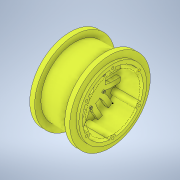
# Autodesk Inventor part: RCT-P009  Rin
Saved by Autodesk Inventor 2020 (Build 240168000, 168)
## iProperties
Created: 2019-09-30
Part Number: RCT-P009  Rin
Material: Genérico
Document SubType Name: Modeling
Designer: david
Density: 1 g/cm^3
Appearance: Valor por defecto
Author: david
Autodesk Inventor part; units mm, degrees
ref_plane "YZ Plane" through (0, 0, 0) normal (1, 0, 0) x (0, 1, 0)
sketch "Boceto1" plane through (0, 0, 0) normal (0, 0, 1) x (1, 0, 0)
  line L0 (0, 0) -> (22.088, 0) construction
  line L1 (12.2099, 0) -> (37.3099, 0) construction
  line L2 (0, 0) -> (0, 21.5) construction
  line L3 (0, 0) -> (21.5, 0) construction
  line L4 (0, 21.5) -> (32.3, 21.5)
  line L5 (0, 21.5) -> (32.3, 21.5) construction
  line L6 (32.3, 21.5) -> (32.3, 28.5)
  line L7 (32.3, 28.5) -> (26.8, 28.5)
  line L8 (0, 21.5) -> (0, 28.5)
  line L9 (0, 21.5) -> (7, 21.5) construction
  line L10 (0, 28.5) -> (5.5, 28.5)
  line L11 (5.5, 28.5) -> (5.5, 24.1)
  line L12 (5.5, 24.1) -> (26.8, 24.1)
  line L13 (26.8, 24.1) -> (26.8, 28.5)
  dimension "d14" = 21.5
  dimension "d15" = 90
  dimension "d16" = 32.3
  dimension "d17" = 0
  dimension "d18" = 7
  dimension "d19" = 5.5
  dimension "d20" = 7
  dimension "d21" = 90
  dimension "d23" = 5.5
  dimension "d24" = 4.4
  constraints: 28 end point, 8 horizontal, 4 perpendicular, 3 equal length, 2 vertical, 1 point on line
  measures "d14" distance of L0.start L2.end
  measures "d15" angle of L3 L2
  measures "d16" distance of L2.end L4.end
  measures "d17" distance between parallel lines of L4 L5
  measures "d18" distance of L4.end L6.end
  measures "d19" distance of L6.end L7.end
  measures "d20" distance of L2.end L8.end
  measures "d21" angle of L9 L8
  measures "d23" distance of L8.end L10.end
  measures "d24" distance of L10.end L11.end
revolve "Revolución1" add sketch "Boceto1" angle 360 about axis through (12.2099, 0, 0) along (1, 0, 0)
ref_plane "Plano de trabajo1" through (16.5, 0, 0) normal (-1, 0, 0) x (0, 0, 1)
sketch "Boceto2" plane through (16.5, 0, 0) normal (-1, 0, 0) x (0, 0, 1)
  point P0 (0, 0)
  point P1 (0, 0)
sketch "Boceto12" plane through (16.5, 0, 0) normal (-1, 0, 0) x (0, 0, 1)
  circle A0 centre (0, 0) radius 10.45
  dimension "d56" = 20.9
  constraints: 1 centre point, 1 coincident
  measures "d56" diameter of A0
extrude "Extrusión10" add sketch "Boceto12" along normal blind 4
sketch "Boceto13" plane through (12.5, 0, 0) normal (-1, 0, 0) x (0, 0, 1)
  circle A0 centre (0, 0) radius 8.8
  dimension "d59" = 17.6
  constraints: 1 centre point, 1 coincident
  measures "d59" diameter of A0
extrude "Extrusión11" add sketch "Boceto13" along normal blind 4.2
sketch "Boceto14" plane through (8.3, 0, 0) normal (-1, 0, 0) x (0, 0, 1)
  line L0 (0, 6.8127) -> (5.9, 3.4064)
  line L1 (5.9, 3.4064) -> (5.9, -3.4064)
  line L2 (5.9, -3.4064) -> (0, -6.8127)
  line L3 (0, -6.8127) -> (-5.9, -3.4064)
  line L4 (-5.9, -3.4064) -> (-5.9, 3.4064)
  line L5 (-5.9, 3.4064) -> (0, 6.8127)
  point P0 (0, 0)
  point P1 (0, 0)
  dimension "d62" = 11.8
  constraints: 12 end point, 1 coincident, 13 other
  measures "d62" distance between parallel lines of L1 L4
extrude "Extrusión12" cut sketch "Boceto14" against normal blind 4
sketch "Boceto15" plane through (12.3, 0, 0) normal (-1, 0, 0) x (0, 0, 1)
  circle A0 centre (0, 0) radius 4.5
  dimension "d65" = 9
  constraints: 1 centre point, 1 coincident
  measures "d65" diameter of A0
extrude "Extrusión13" cut sketch "Boceto15" against normal blind 1
sketch "Boceto16" plane through (13.3, 0, 0) normal (-1, 0, 0) x (0, 0, 1)
  circle A0 centre (0, 0) radius 3.5
  dimension "d68" = 7
  constraints: 1 centre point, 1 coincident
  measures "d68" diameter of A0
extrude "Extrusión14" cut sketch "Boceto16" against normal blind 2.1
sketch "Boceto17" plane through (15.4, 0, 0) normal (-1, 0, 0) x (0, 0, 1)
  circle A0 centre (0, 0) radius 2.5
  dimension "d71" = 5
  constraints: 1 centre point, 1 coincident
  measures "d71" diameter of A0
extrude "Extrusión15" cut sketch "Boceto17" against normal blind 2.1
ref_plane "Plano de trabajo2" through (12.5, 0, 0) normal (-1, 0, 0) x (0, 0, 1)
sketch "Boceto20" plane through (12.5, 0, 0) normal (-1, 0, 0) x (0, 0, 1)
  line L0 (0.0673, 12.0664) -> (10.4835, 5.9749) construction
  line L1 (10.4835, 5.9749) -> (10.4162, -6.0915) construction
  line L2 (10.4162, -6.0915) -> (-0.0673, -12.0664) construction
  line L3 (-0.0673, -12.0664) -> (-10.4835, -5.9749) construction
  line L4 (-10.4835, -5.9749) -> (-10.4162, 6.0915) construction
  line L5 (-10.4162, 6.0915) -> (0.0673, 12.0664) construction
  circle A0 centre (0, 0) radius 10.45
  line L6 (0.0673, 12.0664) -> (-0.9327, 12.0664)
  line L7 (-0.9327, 12.0664) -> (-1.9587, 14.8855)
  circle A1 centre (0, 0) radius 21.5
  line L8 (0, 21.5) -> (0, 20.8746) construction
  line L9 (-1.9587, 14.8855) -> (-5.3823, 20.8154)
  line L10 (-1.9587, 14.8855) -> (4.8885, 14.8855) construction
  line L11 (-8.5615, 19.7218) -> (-4.961, 13.4855)
  line L12 (-4.961, 13.4855) -> (-3.6205, 9.8028)
  line L13 (0, 8.7664) -> (0.0673, 8.7664)
  line L14 (1.9587, 14.8855) -> (5.3823, 20.8154)
  line L15 (0.9327, 12.0664) -> (1.9587, 14.8855)
  line L16 (8.5615, 19.7218) -> (4.961, 13.4855)
  line L17 (4.961, 13.4855) -> (3.6205, 9.8028)
  line L18 (-0.0673, 12.0664) -> (0.9327, 12.0664)
  line L19 (-21.3604, 2.4464) -> (-14.1593, 2.4464)
  line L20 (-14.1593, 2.4464) -> (-10.2997, 1.7659)
  line L21 (-10.9162, 5.2255) -> (-13.8706, 5.7464)
  line L22 (-13.8706, 5.7464) -> (-20.7178, 5.7464)
  line L23 (-10.4162, 6.0915) -> (-10.9162, 5.2255)
  line L24 (-10.4835, 5.9749) -> (-9.9835, 6.8409)
  line L25 (-9.9835, 6.8409) -> (-11.9119, 9.1391)
  line L26 (-11.9119, 9.1391) -> (-15.3355, 15.0689)
  line L27 (-12.7989, 17.2754) -> (-9.1983, 11.0391)
  line L28 (-9.1983, 11.0391) -> (-6.6792, 8.0369)
  line L29 (-12.7989, -17.2754) -> (-9.1983, -11.0391)
  line L30 (-9.1983, -11.0391) -> (-6.6792, -8.0369)
  line L31 (-9.9835, -6.8409) -> (-11.9119, -9.1391)
  line L32 (-11.9119, -9.1391) -> (-15.3355, -15.0689)
  line L33 (-10.4835, -5.9749) -> (-9.9835, -6.8409)
  line L34 (-10.4162, -6.0915) -> (-10.9162, -5.2255)
  line L35 (-10.9162, -5.2255) -> (-13.8706, -5.7464)
  line L36 (-13.8706, -5.7464) -> (-20.7178, -5.7464)
  line L37 (-21.3604, -2.4464) -> (-14.1593, -2.4464)
  line L38 (-14.1593, -2.4464) -> (-10.2997, -1.7659)
  line L39 (8.5615, -19.7218) -> (4.961, -13.4855)
  line L40 (4.961, -13.4855) -> (3.6205, -9.8028)
  line L41 (0.9327, -12.0664) -> (1.9587, -14.8855)
  line L42 (1.9587, -14.8855) -> (5.3823, -20.8154)
  line L43 (-0.0673, -12.0664) -> (0.9327, -12.0664)
  line L44 (0.0673, -12.0664) -> (-0.9327, -12.0664)
  line L45 (-0.9327, -12.0664) -> (-1.9587, -14.8855)
  line L46 (-1.9587, -14.8855) -> (-5.3823, -20.8154)
  line L47 (-8.5615, -19.7218) -> (-4.961, -13.4855)
  line L48 (-4.961, -13.4855) -> (-3.6205, -9.8028)
  line L49 (21.3604, -2.4464) -> (14.1593, -2.4464)
  line L50 (14.1593, -2.4464) -> (10.2997, -1.7659)
  line L51 (10.9162, -5.2255) -> (13.8706, -5.7464)
  line L52 (13.8706, -5.7464) -> (20.7178, -5.7464)
  line L53 (10.4162, -6.0915) -> (10.9162, -5.2255)
  line L54 (10.4835, -5.9749) -> (9.9835, -6.8409)
  line L55 (9.9835, -6.8409) -> (11.9119, -9.1391)
  line L56 (11.9119, -9.1391) -> (15.3355, -15.0689)
  line L57 (12.7989, -17.2754) -> (9.1983, -11.0391)
  line L58 (9.1983, -11.0391) -> (6.6792, -8.0369)
  line L59 (12.7989, 17.2754) -> (9.1983, 11.0391)
  line L60 (9.1983, 11.0391) -> (6.6792, 8.0369)
  line L61 (9.9835, 6.8409) -> (11.9119, 9.1391)
  line L62 (11.9119, 9.1391) -> (15.3355, 15.0689)
  line L63 (10.4835, 5.9749) -> (9.9835, 6.8409)
  line L64 (10.4162, 6.0915) -> (10.9162, 5.2255)
  line L65 (10.9162, 5.2255) -> (13.8706, 5.7464)
  line L66 (13.8706, 5.7464) -> (20.7178, 5.7464)
  line L67 (21.3604, 2.4464) -> (14.1593, 2.4464)
  line L68 (14.1593, 2.4464) -> (10.2997, 1.7659)
  arc A2 (21.3604, 2.4464) -> (12.7989, 17.2754) centre (0, 0) ccw
  arc A3 (8.5615, 19.7218) -> (-8.5615, 19.7218) centre (0, 0) ccw
  arc A4 (-12.7989, 17.2754) -> (-21.3604, 2.4464) centre (0, 0) ccw
  arc A5 (-21.3604, -2.4464) -> (-12.7989, -17.2754) centre (0, 0) ccw
  arc A6 (-21.3604, -2.4464) -> (-12.7989, -17.2754) centre (0, 0) ccw
  arc A7 (-12.7989, 17.2754) -> (-21.3604, 2.4464) centre (0, 0) ccw
  arc A8 (8.5615, 19.7218) -> (-8.5615, 19.7218) centre (0, 0) ccw
  arc A9 (21.3604, 2.4464) -> (12.7989, 17.2754) centre (0, 0) ccw
  arc A10 (-8.5615, -19.7218) -> (8.5615, -19.7218) centre (0, 0) ccw
  arc A11 (12.7989, -17.2754) -> (21.3604, -2.4464) centre (0, 0) ccw
  arc A12 (-8.5615, -19.7218) -> (8.5615, -19.7218) centre (0, 0) ccw
  arc A13 (12.7989, -17.2754) -> (21.3604, -2.4464) centre (0, 0) ccw
  arc A14 (3.6205, 9.8028) -> (-3.6205, 9.8028) centre (0, 0) ccw
  arc A15 (-6.6792, 8.0369) -> (-10.2997, 1.7659) centre (0, 0) ccw
  arc A16 (-10.2997, -1.7659) -> (-6.6792, -8.0369) centre (0, 0) ccw
  arc A17 (-3.6205, -9.8028) -> (3.6205, -9.8028) centre (0, 0) ccw
  arc A18 (6.6792, -8.0369) -> (10.2997, -1.7659) centre (0, 0) ccw
  arc A19 (10.2997, 1.7659) -> (6.6792, 8.0369) centre (0, 0) ccw
  dimension "d107" = 1
  dimension "d108" = 3
  dimension "d109" = 120
  dimension "d110" = 3.3
  dimension "d111" = 360
  dimension "d114" = 5.9299
  dimension "d115" = 3.02
  constraints: 138 end point, 38 point on circle, 19 centre point, 7 symmetric about line, 4 coincident, 3 parallel, 2 horizontal, 1 concentric, 1 equal length, 1 point on line, 1 vertical, 163 other
  measures "d107" distance of L6.start L6.end
  measures "d108" distance of L6.end L10.start
  measures "d109" angle of L10 L9
  measures "d110" distance between parallel lines of L9 L11
  measures "d114" vertical distance of L14.start L14.end
  measures "d115" distance from line of L13.end L66
extrude "Extrusión16" add sketch "Boceto20" against normal blind 4 contours A0 L60 L59 A1 L62 L61 L63 L64 L65 L66 L67 L68 | L50 L49 A1 L52 L51 L53 L54 L55 L56 L57 L58 A0 | A0 L12 L11 A1 L9 L7 L6 L18 L15 L14 L16 L17 | L40 L39 A1 L42 L41 L43 L44 L45 L46 L47 L48 A0 | L66 L65 L64 L63 L61 L62 A1 | A1 L56 L55 L54 L53 L51 L52 | A0 L20 L19 A1 L22 L21 L23 L24 L25 L26 L27 L28 | L30 L29 A1 L32 L31 L33 L34 L35 L36 L37 L38 A0 | L14 L15 L18 L6 L7 L9 A1 | A1 L46 L45 L44 L43 L41 L42 | L26 L25 L24 L23 L21 L22 A1 | A1 L36 L35 L34 L33 L31 L32
sketch "Boceto22" plane through (16.5, 0, 0) normal (1, 0, 0) x (0, 0, -1)
  line L0 (1.9587, 14.8855) -> (5.3823, 20.8154)
  line L1 (0.9327, 12.0664) -> (1.9587, 14.8855)
  line L2 (-0.0673, 12.0664) -> (0.9327, 12.0664)
  line L3 (0, 21.5) -> (0, 20.8746) construction
  line L4 (0.0673, 12.0664) -> (-0.9327, 12.0664)
  line L5 (-1.9587, 14.8855) -> (4.8885, 14.8855) construction
  line L6 (-0.9327, 12.0664) -> (-1.9587, 14.8855)
  line L7 (-1.9587, 14.8855) -> (-5.3823, 20.8154)
  arc A0 (5.3823, 20.8154) -> (-5.3823, 20.8154) centre (0, 0) ccw
  circle A1 centre (0, 0) radius 21.5 projected
  line L8 (-5.3823, 20.8154) -> (-1.9587, 14.8855)
  line L9 (-0.9327, 12.0664) -> (0.9327, 12.0664)
  line L10 (1.9587, 14.8855) -> (5.3823, 20.8154)
  line L11 (-10.4835, 5.9749) -> (-9.9835, 6.8409)
  line L12 (-10.4162, 6.0915) -> (-10.9162, 5.2255)
  line L13 (-10.9162, 5.2255) -> (-9.9835, 6.8409)
  line L14 (-9.9835, 6.8409) -> (-11.9119, 9.1391)
  line L15 (-10.9162, 5.2255) -> (-13.8706, 5.7464)
  line L16 (-13.8706, 5.7464) -> (-10.447, 11.6763) construction
  line L17 (-11.9119, 9.1391) -> (-15.3355, 15.0689)
  line L18 (-11.9119, 9.1391) -> (-15.3355, 15.0689)
  line L19 (-13.8706, 5.7464) -> (-20.7178, 5.7464)
  line L20 (-20.7178, 5.7464) -> (-13.8706, 5.7464)
  arc A2 (-15.3355, 15.0689) -> (-20.7178, 5.7464) centre (0, 0) ccw
  line L21 (-18.6195, 10.75) -> (-18.0779, 10.4373) construction
  line L22 (-10.4162, -6.0915) -> (-10.9162, -5.2255)
  line L23 (-10.4835, -5.9749) -> (-9.9835, -6.8409)
  line L24 (-9.9835, -6.8409) -> (-10.9162, -5.2255)
  line L25 (-10.9162, -5.2255) -> (-13.8706, -5.7464)
  line L26 (-9.9835, -6.8409) -> (-11.9119, -9.1391)
  line L27 (-11.9119, -9.1391) -> (-15.3355, -3.2092) construction
  line L28 (-13.8706, -5.7464) -> (-20.7178, -5.7464)
  line L29 (-13.8706, -5.7464) -> (-20.7178, -5.7464)
  line L30 (-11.9119, -9.1391) -> (-15.3355, -15.0689)
  line L31 (-15.3355, -15.0689) -> (-11.9119, -9.1391)
  arc A3 (-20.7178, -5.7464) -> (-15.3355, -15.0689) centre (0, 0) ccw
  line L32 (-18.6195, -10.75) -> (-18.0779, -10.4373) construction
  line L33 (0.0673, -12.0664) -> (-0.9327, -12.0664)
  line L34 (-0.0673, -12.0664) -> (0.9327, -12.0664)
  line L35 (0.9327, -12.0664) -> (-0.9327, -12.0664)
  line L36 (-0.9327, -12.0664) -> (-1.9587, -14.8855)
  line L37 (0.9327, -12.0664) -> (1.9587, -14.8855)
  line L38 (1.9587, -14.8855) -> (-4.8885, -14.8855) construction
  line L39 (-1.9587, -14.8855) -> (-5.3823, -20.8154)
  line L40 (-1.9587, -14.8855) -> (-5.3823, -20.8154)
  line L41 (1.9587, -14.8855) -> (5.3823, -20.8154)
  line L42 (5.3823, -20.8154) -> (1.9587, -14.8855)
  arc A4 (-5.3823, -20.8154) -> (5.3823, -20.8154) centre (0, 0) ccw
  line L43 (0, -21.5) -> (0, -20.8746) construction
  line L44 (10.4835, -5.9749) -> (9.9835, -6.8409)
  line L45 (10.4162, -6.0915) -> (10.9162, -5.2255)
  line L46 (10.9162, -5.2255) -> (9.9835, -6.8409)
  line L47 (9.9835, -6.8409) -> (11.9119, -9.1391)
  line L48 (10.9162, -5.2255) -> (13.8706, -5.7464)
  line L49 (13.8706, -5.7464) -> (10.447, -11.6763) construction
  line L50 (11.9119, -9.1391) -> (15.3355, -15.0689)
  line L51 (11.9119, -9.1391) -> (15.3355, -15.0689)
  line L52 (13.8706, -5.7464) -> (20.7178, -5.7464)
  line L53 (20.7178, -5.7464) -> (13.8706, -5.7464)
  arc A5 (15.3355, -15.0689) -> (20.7178, -5.7464) centre (0, 0) ccw
  line L54 (18.6195, -10.75) -> (18.0779, -10.4373) construction
  line L55 (10.4162, 6.0915) -> (10.9162, 5.2255)
  line L56 (10.4835, 5.9749) -> (9.9835, 6.8409)
  line L57 (9.9835, 6.8409) -> (10.9162, 5.2255)
  line L58 (10.9162, 5.2255) -> (13.8706, 5.7464)
  line L59 (9.9835, 6.8409) -> (11.9119, 9.1391)
  line L60 (11.9119, 9.1391) -> (15.3355, 3.2092) construction
  line L61 (13.8706, 5.7464) -> (20.7178, 5.7464)
  line L62 (13.8706, 5.7464) -> (20.7178, 5.7464)
  line L63 (11.9119, 9.1391) -> (15.3355, 15.0689)
  line L64 (15.3355, 15.0689) -> (11.9119, 9.1391)
  arc A6 (20.7178, 5.7464) -> (15.3355, 15.0689) centre (0, 0) ccw
  line L65 (18.6195, 10.75) -> (18.0779, 10.4373) construction
  point P0 (4.961, 13.4855)
  point P1 (0, 8.7664)
  point P2 (-4.961, 13.4855)
  point P3 (-7.592, 4.3832)
  point P4 (-9.1983, 11.0391)
  point P5 (-14.1593, 2.4464)
  point P6 (-7.592, -4.3832)
  point P7 (-14.1593, -2.4464)
  point P8 (-9.1983, -11.0391)
  point P9 (0, -8.7664)
  point P10 (-4.961, -13.4855)
  point P11 (4.961, -13.4855)
  point P12 (7.592, -4.3832)
  point P13 (9.1983, -11.0391)
  point P14 (14.1593, -2.4464)
  point P15 (7.592, 4.3832)
  point P16 (14.1593, 2.4464)
  point P17 (9.1983, 11.0391)
  dimension "d116" = 1
  dimension "d117" = 3
  dimension "d118" = 120
  dimension "d119" = 5.9299
  dimension "d120" = 170
  dimension "d121" = 5.3823
  dimension "d122" = 3.3
  dimension "d123" = 1.4
  dimension "d124" = 5.0036
  dimension "d125" = 4.6908
  dimension "d126" = 1.3632
  dimension "d129" = 360
  constraints: 132 end point, 12 point on circle, 6 centre point, 6 point on line, 5 symmetric about line, 3 horizontal, 1 coincident, 1 collinear, 1 concentric, 1 equal length, 1 parallel, 1 vertical, 163 other
  measures "d116" distance of L4.start L4.end
  measures "d117" distance of L4.end L5.start
  measures "d118" angle of L5 L7
  measures "d119" vertical distance of L1.end L0.end
  measures "d120" angle of L1 L10
  measures "d121" distance from line of L0.end L3
  measures "d122" distance from line of point (4.961, 13.486) L10
  measures "d123" distance from line of point (4.961, 13.486) L5
  measures "d124" distance from line of L3.start L10
  measures "d125" distance from line of L3.end L10
  measures "d126" distance from line of point (0, 8.766) L10
extrude "Extrusión17" cut sketch "Boceto22" against normal blind 2 contours L1 L2 L4 L6 L7 A0 L0 | A1 L61 L58 L55 L56 L59 L63 | L17 L14 L11 L12 L15 L19 A1 | L28 L25 L22 L23 L26 L30 A1 | A1 L50 L47 L44 L45 L48 L52 | L39 L36 L33 L34 L37 L41 A1
sketch "Boceto23" plane through (32.3, 0, 0) normal (1, 0, 0) x (0, 0, -1)
  circle A0 centre (0, 0) radius 28.5
  circle A1 centre (0, 0) radius 26
  circle A2 centre (0, 0) radius 24
  dimension "d133" = 2.5
  dimension "d134" = 2
  dimension "d135" = 57
  constraints: 3 centre point, 1 coincident
  measures "d133" radial gap between concentric circles of A0 A1
  measures "d134" radial gap between concentric circles of A1 A2
  measures "d135" diameter of A0
extrude "Extrusión18" cut sketch "Boceto23" against normal blind 2 contours A1
sketch "Boceto24" plane through (0, 0, 0) normal (-1, 0, 0) x (0, 0, 1)
  circle A0 centre (0, 0) radius 28.5
  circle A1 centre (0, 0) radius 28.5 projected
  circle A2 centre (0, 0) radius 26
  circle A3 centre (0, 0) radius 24
  dimension "d138" = 2.5
  dimension "d139" = 2
  constraints: 3 centre point, 1 coincident, 1 concentric
  measures "d138" radial gap between concentric circles of A0 A2
  measures "d139" radial gap between concentric circles of A2 A3
extrude "Extrusión19" cut sketch "Boceto24" against normal blind 2 contours A2
sketch "Boceto28" plane through (12.5, 0, 0) normal (-1, 0, 0) x (0, 0, 1)
  line L0 (8.5615, -19.7218) -> (4.961, -13.4855)
  line L1 (4.961, -13.4855) -> (3.6205, -9.8028)
  line L2 (-0.0673, -12.0664) -> (0.9327, -12.0664)
  line L3 (0.0673, -12.0664) -> (-0.9327, -12.0664)
  line L4 (0.9327, -12.0664) -> (1.9587, -14.8855)
  arc A0 (-3.6205, -9.8028) -> (3.6205, -9.8028) centre (0, 0) ccw
  line L5 (-0.9327, -12.0664) -> (-1.9587, -14.8855)
  line L6 (-4.961, -13.4855) -> (-3.6205, -9.8028)
  line L7 (1.9587, -14.8855) -> (5.3823, -20.8154)
  line L8 (-1.9587, -14.8855) -> (-5.3823, -20.8154)
  line L9 (-8.5615, -19.7218) -> (-4.961, -13.4855)
  line L10 (4.961, -13.4855) -> (8.5615, -19.7218) projected
  line L11 (3.6205, -9.8028) -> (4.961, -13.4855) projected
  line L12 (8.5615, -19.7218) -> (4.961, -13.4855)
  line L13 (4.961, -13.4855) -> (3.6205, -9.8028)
  arc A1 (-5.3823, -20.8154) -> (5.3823, -20.8154) centre (0, 0) ccw projected
  line L14 (5.3823, -20.8154) -> (1.9587, -14.8855)
  line L15 (1.9587, -14.8855) -> (0.9327, -12.0664) projected
  line L16 (0.9327, -12.0664) -> (-0.9327, -12.0664)
  line L17 (-1.9587, -14.8855) -> (-5.3823, -20.8154)
  line L18 (-8.5615, -19.7218) -> (-4.961, -13.4855)
  arc A2 (-3.6205, -9.8028) -> (3.6205, -9.8028) centre (0, 0) ccw
  circle A3 centre (0, 0) radius 21.5 projected
  arc A4 (-8.5615, -19.7218) -> (-5.3823, -20.8154) centre (0, 0) ccw
  arc A5 (5.3823, -20.8154) -> (8.5615, -19.7218) centre (0, 0) ccw
  arc A6 (-8.5615, -19.7218) -> (-5.3823, -20.8154) centre (0, 0) ccw
  arc A7 (5.3823, -20.8154) -> (8.5615, -19.7218) centre (0, 0) ccw
  arc A8 (5.3823, -20.8154) -> (8.5615, -19.7218) centre (0, 0) ccw
  arc A9 (-8.5615, -19.7218) -> (-5.3823, -20.8154) centre (0, 0) ccw
  arc A10 (-6.6792, -8.0369) -> (-3.6205, -9.8028) centre (0, 0) ccw projected
  line L19 (-4.961, -13.4855) -> (-3.6205, -9.8028) projected
  line L20 (-3.6205, -9.8028) -> (-4.961, -13.4855)
  line L21 (-8.5615, -19.7218) -> (-4.961, -13.4855) projected
  line L22 (-4.961, -13.4855) -> (-8.5615, -19.7218)
  line L23 (10.4835, -5.9749) -> (9.9835, -6.8409)
  line L24 (10.4162, -6.0915) -> (10.9162, -5.2255)
  line L25 (10.9162, -5.2255) -> (9.9835, -6.8409)
  line L26 (9.1983, -11.0391) -> (6.6792, -8.0369)
  line L27 (6.6792, -8.0369) -> (9.1983, -11.0391)
  arc A11 (6.6792, -8.0369) -> (10.2997, -1.7659) centre (0, 0) ccw
  arc A12 (6.6792, -8.0369) -> (10.2997, -1.7659) centre (0, 0) ccw
  line L28 (9.9835, -6.8409) -> (11.9119, -9.1391)
  line L29 (10.9162, -5.2255) -> (13.8706, -5.7464)
  line L30 (14.1593, -2.4464) -> (10.2997, -1.7659)
  line L31 (13.8706, -5.7464) -> (20.7178, -5.7464)
  line L32 (20.7178, -5.7464) -> (13.8706, -5.7464)
  line L33 (21.3604, -2.4464) -> (14.1593, -2.4464)
  line L34 (21.3604, -2.4464) -> (14.1593, -2.4464)
  line L35 (14.1593, -2.4464) -> (10.2997, -1.7659)
  line L36 (11.9119, -9.1391) -> (15.3355, -15.0689)
  line L37 (11.9119, -9.1391) -> (15.3355, -15.0689)
  line L38 (12.7989, -17.2754) -> (9.1983, -11.0391)
  line L39 (9.1983, -11.0391) -> (12.7989, -17.2754)
  arc A13 (12.7989, -17.2754) -> (15.3355, -15.0689) centre (0, 0) ccw
  line L40 (12.7989, -17.2754) -> (9.1983, -11.0391)
  arc A14 (20.7178, -5.7464) -> (21.3604, -2.4464) centre (0, 0) ccw
  arc A15 (12.7989, -17.2754) -> (15.3355, -15.0689) centre (0, 0) ccw
  arc A16 (12.7989, -17.2754) -> (15.3355, -15.0689) centre (0, 0) ccw
  arc A17 (20.7178, -5.7464) -> (21.3604, -2.4464) centre (0, 0) ccw
  arc A18 (20.7178, -5.7464) -> (21.3604, -2.4464) centre (0, 0) ccw
  line L41 (10.4162, 6.0915) -> (10.9162, 5.2255)
  line L42 (10.4835, 5.9749) -> (9.9835, 6.8409)
  line L43 (9.9835, 6.8409) -> (10.9162, 5.2255)
  line L44 (14.1593, 2.4464) -> (10.2997, 1.7659)
  line L45 (10.2997, 1.7659) -> (14.1593, 2.4464)
  arc A19 (10.2997, 1.7659) -> (6.6792, 8.0369) centre (0, 0) ccw
  arc A20 (10.2997, 1.7659) -> (6.6792, 8.0369) centre (0, 0) ccw
  line L46 (10.9162, 5.2255) -> (13.8706, 5.7464)
  line L47 (9.9835, 6.8409) -> (11.9119, 9.1391)
  line L48 (9.1983, 11.0391) -> (6.6792, 8.0369)
  line L49 (11.9119, 9.1391) -> (15.3355, 15.0689)
  line L50 (15.3355, 15.0689) -> (11.9119, 9.1391)
  line L51 (12.7989, 17.2754) -> (9.1983, 11.0391)
  line L52 (12.7989, 17.2754) -> (9.1983, 11.0391)
  line L53 (9.1983, 11.0391) -> (6.6792, 8.0369)
  line L54 (13.8706, 5.7464) -> (20.7178, 5.7464)
  line L55 (13.8706, 5.7464) -> (20.7178, 5.7464)
  line L56 (21.3604, 2.4464) -> (14.1593, 2.4464)
  line L57 (14.1593, 2.4464) -> (21.3604, 2.4464)
  arc A21 (21.3604, 2.4464) -> (20.7178, 5.7464) centre (0, 0) ccw
  line L58 (21.3604, 2.4464) -> (14.1593, 2.4464)
  arc A22 (15.3355, 15.0689) -> (12.7989, 17.2754) centre (0, 0) ccw
  arc A23 (21.3604, 2.4464) -> (20.7178, 5.7464) centre (0, 0) ccw
  arc A24 (21.3604, 2.4464) -> (20.7178, 5.7464) centre (0, 0) ccw
  arc A25 (15.3355, 15.0689) -> (12.7989, 17.2754) centre (0, 0) ccw
  arc A26 (15.3355, 15.0689) -> (12.7989, 17.2754) centre (0, 0) ccw
  line L59 (-0.0673, 12.0664) -> (0.9327, 12.0664)
  line L60 (0.0673, 12.0664) -> (-0.9327, 12.0664)
  line L61 (-0.9327, 12.0664) -> (0.9327, 12.0664)
  line L62 (4.961, 13.4855) -> (3.6205, 9.8028)
  line L63 (3.6205, 9.8028) -> (4.961, 13.4855)
  arc A27 (3.6205, 9.8028) -> (-3.6205, 9.8028) centre (0, 0) ccw
  arc A28 (3.6205, 9.8028) -> (-3.6205, 9.8028) centre (0, 0) ccw
  line L64 (0.9327, 12.0664) -> (1.9587, 14.8855)
  line L65 (-0.9327, 12.0664) -> (-1.9587, 14.8855)
  line L66 (-4.961, 13.4855) -> (-3.6205, 9.8028)
  line L67 (-1.9587, 14.8855) -> (-5.3823, 20.8154)
  line L68 (-5.3823, 20.8154) -> (-1.9587, 14.8855)
  line L69 (-8.5615, 19.7218) -> (-4.961, 13.4855)
  line L70 (-8.5615, 19.7218) -> (-4.961, 13.4855)
  line L71 (-4.961, 13.4855) -> (-3.6205, 9.8028)
  line L72 (1.9587, 14.8855) -> (5.3823, 20.8154)
  line L73 (1.9587, 14.8855) -> (5.3823, 20.8154)
  line L74 (8.5615, 19.7218) -> (4.961, 13.4855)
  line L75 (4.961, 13.4855) -> (8.5615, 19.7218)
  arc A29 (8.5615, 19.7218) -> (5.3823, 20.8154) centre (0, 0) ccw
  line L76 (8.5615, 19.7218) -> (4.961, 13.4855)
  arc A30 (-5.3823, 20.8154) -> (-8.5615, 19.7218) centre (0, 0) ccw
  arc A31 (8.5615, 19.7218) -> (5.3823, 20.8154) centre (0, 0) ccw
  arc A32 (8.5615, 19.7218) -> (5.3823, 20.8154) centre (0, 0) ccw
  arc A33 (-5.3823, 20.8154) -> (-8.5615, 19.7218) centre (0, 0) ccw
  arc A34 (-5.3823, 20.8154) -> (-8.5615, 19.7218) centre (0, 0) ccw
  line L77 (-10.4835, 5.9749) -> (-9.9835, 6.8409)
  line L78 (-10.4162, 6.0915) -> (-10.9162, 5.2255)
  line L79 (-10.9162, 5.2255) -> (-9.9835, 6.8409)
  line L80 (-9.1983, 11.0391) -> (-6.6792, 8.0369)
  line L81 (-6.6792, 8.0369) -> (-9.1983, 11.0391)
  arc A35 (-6.6792, 8.0369) -> (-10.2997, 1.7659) centre (0, 0) ccw
  arc A36 (-6.6792, 8.0369) -> (-10.2997, 1.7659) centre (0, 0) ccw
  line L82 (-9.9835, 6.8409) -> (-11.9119, 9.1391)
  line L83 (-10.9162, 5.2255) -> (-13.8706, 5.7464)
  line L84 (-14.1593, 2.4464) -> (-10.2997, 1.7659)
  line L85 (-13.8706, 5.7464) -> (-20.7178, 5.7464)
  line L86 (-20.7178, 5.7464) -> (-13.8706, 5.7464)
  line L87 (-21.3604, 2.4464) -> (-14.1593, 2.4464)
  line L88 (-21.3604, 2.4464) -> (-14.1593, 2.4464)
  line L89 (-14.1593, 2.4464) -> (-10.2997, 1.7659)
  line L90 (-11.9119, 9.1391) -> (-15.3355, 15.0689)
  line L91 (-11.9119, 9.1391) -> (-15.3355, 15.0689)
  line L92 (-12.7989, 17.2754) -> (-9.1983, 11.0391)
  line L93 (-9.1983, 11.0391) -> (-12.7989, 17.2754)
  arc A37 (-12.7989, 17.2754) -> (-15.3355, 15.0689) centre (0, 0) ccw
  line L94 (-12.7989, 17.2754) -> (-9.1983, 11.0391)
  arc A38 (-20.7178, 5.7464) -> (-21.3604, 2.4464) centre (0, 0) ccw
  arc A39 (-12.7989, 17.2754) -> (-15.3355, 15.0689) centre (0, 0) ccw
  arc A40 (-12.7989, 17.2754) -> (-15.3355, 15.0689) centre (0, 0) ccw
  arc A41 (-20.7178, 5.7464) -> (-21.3604, 2.4464) centre (0, 0) ccw
  arc A42 (-20.7178, 5.7464) -> (-21.3604, 2.4464) centre (0, 0) ccw
  line L95 (-10.4162, -6.0915) -> (-10.9162, -5.2255)
  line L96 (-10.4835, -5.9749) -> (-9.9835, -6.8409)
  line L97 (-9.9835, -6.8409) -> (-10.9162, -5.2255)
  line L98 (-14.1593, -2.4464) -> (-10.2997, -1.7659)
  line L99 (-10.2997, -1.7659) -> (-14.1593, -2.4464)
  arc A43 (-10.2997, -1.7659) -> (-6.6792, -8.0369) centre (0, 0) ccw
  arc A44 (-10.2997, -1.7659) -> (-6.6792, -8.0369) centre (0, 0) ccw
  line L100 (-10.9162, -5.2255) -> (-13.8706, -5.7464)
  line L101 (-9.9835, -6.8409) -> (-11.9119, -9.1391)
  line L102 (-9.1983, -11.0391) -> (-6.6792, -8.0369)
  line L103 (-11.9119, -9.1391) -> (-15.3355, -15.0689)
  line L104 (-15.3355, -15.0689) -> (-11.9119, -9.1391)
  line L105 (-12.7989, -17.2754) -> (-9.1983, -11.0391)
  line L106 (-12.7989, -17.2754) -> (-9.1983, -11.0391)
  line L107 (-9.1983, -11.0391) -> (-6.6792, -8.0369)
  line L108 (-13.8706, -5.7464) -> (-20.7178, -5.7464)
  line L109 (-13.8706, -5.7464) -> (-20.7178, -5.7464)
  line L110 (-21.3604, -2.4464) -> (-14.1593, -2.4464)
  line L111 (-14.1593, -2.4464) -> (-21.3604, -2.4464)
  arc A45 (-21.3604, -2.4464) -> (-20.7178, -5.7464) centre (0, 0) ccw
  line L112 (-21.3604, -2.4464) -> (-14.1593, -2.4464)
  arc A46 (-15.3355, -15.0689) -> (-12.7989, -17.2754) centre (0, 0) ccw
  arc A47 (-21.3604, -2.4464) -> (-20.7178, -5.7464) centre (0, 0) ccw
  arc A48 (-21.3604, -2.4464) -> (-20.7178, -5.7464) centre (0, 0) ccw
  arc A49 (-15.3355, -15.0689) -> (-12.7989, -17.2754) centre (0, 0) ccw
  arc A50 (-15.3355, -15.0689) -> (-12.7989, -17.2754) centre (0, 0) ccw
  point P0 (-0.0673, -12.0664)
  point P1 (9.1983, -11.0391)
  point P2 (10.4162, -6.0915)
  point P3 (14.1593, 2.4464)
  point P4 (10.4835, 5.9749)
  point P5 (4.961, 13.4855)
  point P6 (0.0673, 12.0664)
  point P7 (-9.1983, 11.0391)
  point P8 (-10.4162, 6.0915)
  point P9 (-14.1593, -2.4464)
  point P10 (-10.4835, -5.9749)
  point P11 (-4.961, -13.4855)
  dimension "d153" = 360
  constraints: 216 end point, 96 point on circle, 48 centre point, 19 coincident, 4 collinear, 1 concentric, 1 horizontal, 283 other
extrude "Extrusión20" cut sketch "Boceto28" against normal blind 1 contours A3 L7 L4 L2 L3 L5 L8 L9 L6 A0 L1 L0 | L38 L26 A11 L30 L33 A3 L31 L29 L24 L23 L28 L36 | L102 L105 A3 L103 L101 L96 L95 L100 L108 L110 L98 A43 | L56 L44 A19 L48 L51 A3 L49 L47 L42 L41 L46 L54 | A3 L85 L83 L78 L77 L82 L90 L92 L80 A35 L84 L87 | L74 L62 A27 L66 L69 A3 L67 L65 L60 L59 L64 L72
sketch "Boceto31" plane through (16.5, 0, 0) normal (1, 0, 0) x (0, 0, -1)
  circle A0 centre (0, 0) radius 8.8
  line L0 (10.9162, -5.2255) -> (10.4162, -6.0915) construction
  line L1 (9.9835, -6.8409) -> (10.9162, -5.2255) construction
  circle A1 centre (0, 0) radius 8.8 construction
  line L2 (10.4162, -6.0915) -> (7.5871, -4.4582) construction
  line L3 (10.4162, -6.0915) -> (9.0015, -5.2748) construction
  circle A2 centre (9.0015, -5.2748) radius 1
  circle A3 centre (9.0688, 5.1582) radius 1
  circle A4 centre (0.0673, 10.4329) radius 1
  circle A5 centre (-9.0015, 5.2748) radius 1
  circle A6 centre (-9.0688, -5.1582) radius 1
  circle A7 centre (-0.0673, -10.4329) radius 1
  dimension "d174" = 1
  dimension "d175" = 1.6335
  dimension "d176" = 2
  dimension "d177" = 360
  constraints: 8 end point, 7 centre point, 2 coincident, 2 point on line, 16 other
  measures "d174" distance of L0.start L0.end
  measures "d175" distance of L0.end L3.end
  measures "d176" diameter of A2
extrude "Extrusión23" add sketch "Boceto31" along normal blind 0.5 contours A2 | A3 | A4 | A5 | A6 | A7
sketch "Boceto32" plane through (17, -10.4329, 0.0673) normal (1, 0, 0) x (0, 0, -1)
  arc A0 (-3.5532, 0.6302) -> (3.6879, 0.6302) centre (0.0673, 10.4329) ccw projected
  line L0 (0.4262, 0.6302) -> (0.8073, -0.0043)
  line L1 (0.8073, -0.0043) -> (0.4484, -0.6515)
  line L2 (0.4484, -0.6515) -> (-0.2916, -0.6643)
  line L3 (-0.2916, -0.6643) -> (-0.6726, -0.0299)
  line L4 (-0.6726, -0.0299) -> (-0.3137, 0.6174)
  line L5 (-0.3137, 0.6174) -> (0.4262, 0.6302)
  line L6 (8.7584, 4.5607) -> (8.3773, 5.1951)
  line L7 (8.3773, 5.1951) -> (8.7362, 5.8424)
  line L8 (8.7362, 5.8424) -> (9.4762, 5.8552)
  line L9 (9.4762, 5.8552) -> (9.8573, 5.2207)
  line L10 (9.8573, 5.2207) -> (9.4984, 4.5735)
  line L11 (9.4984, 4.5735) -> (8.7584, 4.5607)
  line L12 (9.4984, 15.0235) -> (8.7584, 15.0107)
  line L13 (8.7584, 15.0107) -> (8.3773, 15.6451)
  line L14 (8.3773, 15.6451) -> (8.7362, 16.2924)
  line L15 (8.7362, 16.2924) -> (9.4762, 16.3052)
  line L16 (9.4762, 16.3052) -> (9.8573, 15.6707)
  line L17 (9.8573, 15.6707) -> (9.4984, 15.0235)
  line L18 (0.8073, 20.8957) -> (0.4484, 20.2485)
  line L19 (0.4484, 20.2485) -> (-0.2916, 20.2357)
  line L20 (-0.2916, 20.2357) -> (-0.6726, 20.8701)
  line L21 (-0.6726, 20.8701) -> (-0.3137, 21.5174)
  line L22 (-0.3137, 21.5174) -> (0.4262, 21.5302)
  line L23 (0.4262, 21.5302) -> (0.8073, 20.8957)
  line L24 (-8.6237, 16.3052) -> (-8.2427, 15.6707)
  line L25 (-8.2427, 15.6707) -> (-8.6016, 15.0235)
  line L26 (-8.6016, 15.0235) -> (-9.3415, 15.0107)
  line L27 (-9.3415, 15.0107) -> (-9.7226, 15.6451)
  line L28 (-9.7226, 15.6451) -> (-9.3637, 16.2924)
  line L29 (-9.3637, 16.2924) -> (-8.6237, 16.3052)
  line L30 (-9.3637, 5.8424) -> (-8.6237, 5.8552)
  line L31 (-8.6237, 5.8552) -> (-8.2427, 5.2207)
  line L32 (-8.2427, 5.2207) -> (-8.6016, 4.5735)
  line L33 (-8.6016, 4.5735) -> (-9.3415, 4.5607)
  line L34 (-9.3415, 4.5607) -> (-9.7226, 5.1951)
  line L35 (-9.7226, 5.1951) -> (-9.3637, 5.8424)
  point P0 (0.0673, -0.0171)
  dimension "d182" = 360
  constraints: 72 end point, 1 point on circle, 86 other
extrude "Extrusión24" add sketch "Boceto32" along normal blind 0.5
fillet "Empalme1" radius 0.2 25 edges at (17.5, -9.8092, 0.0111) (17.5, -4.5842, -9.0389) (17.5, -5.5358, -9.6105) (17.5, -5.8658, -9.0611) (17.5, -5.555, -8.5005) (17.5, -4.9142, -8.4894) (17.5, -10.12, -0.5494) (17.5, -10.7608, -0.5605) (17.5, -11.0908, -0.0111) (17.5, -10.78, 0.5494) (17.5, -10.1392, 0.5605) (17.5, -4.895, -9.5994) (17.5, -4.895, 8.5005) (17.5, -5.555, 9.5994) (17.5, -4.9142, 9.6105) (17.5, -5.8658, 9.0389) (17.5, -5.5358, 8.4894) (17.5, -4.5842, 9.0611) (17.5, 5.555, 8.5005) (17.5, 4.895, 9.5994) (17.5, 5.8658, 9.0611) (17.5, 5.5358, 9.6105) (17.5, 4.5842, 9.0389) (17.25, 5.2378, 8.31) (17.5, 4.9142, 8.4894)
fillet "Empalme2" radius 0.2 12 edges at (17.5, 10.78, -0.5494) (17.5, 11.0908, 0.0111) (17.5, 10.7608, 0.5605) (17.5, 10.12, 0.5494) (17.5, 9.8092, -0.0111) (17.5, 10.1392, -0.5605) (17.5, 5.555, -9.5994) (17.5, 5.8658, -9.0389) (17.5, 5.5358, -8.4894) (17.5, 4.895, -8.5005) (17.5, 4.5842, -9.0611) (17.5, 4.9142, -9.6105)
sketch "Boceto33" plane through (32.3, 0, 0) normal (1, 0, 0) x (0, 0, -1)
  circle A0 centre (0, 0) radius 21.5 projected
  circle A1 centre (0, -21.5) radius 2.25
  circle A2 centre (0, -21.5) radius 0.85
  circle A3 centre (18.6195, -10.75) radius 2.25
  circle A4 centre (18.6195, -10.75) radius 0.85
  circle A5 centre (18.6195, 10.75) radius 2.25
  circle A6 centre (18.6195, 10.75) radius 0.85
  circle A7 centre (0, 21.5) radius 2.25
  circle A8 centre (0, 21.5) radius 0.85
  circle A9 centre (-18.6195, 10.75) radius 2.25
  circle A10 centre (-18.6195, 10.75) radius 0.85
  circle A11 centre (-18.6195, -10.75) radius 2.25
  circle A12 centre (-18.6195, -10.75) radius 0.85
  dimension "d188" = 4.5
  dimension "d189" = 1.7
  dimension "d192" = 360
  constraints: 12 centre point, 6 coincident, 1 vertical alignment, 26 other
  measures "d188" diameter of A1
  measures "d189" diameter of A2
extrude "Extrusión25" add sketch "Boceto33" against normal blind 32.3 contours A5 A0 A6 | A0 A6 A5 | A3 A0 A4 | A0 A4 A3 | A7 A0 A8 | A0 A8 A7 | A1 A0 A2 | A0 A2 A1 | A9 A0 A10 | A0 A10 A9 | A11 A0 A12 | A0 A12 A11
extrude "Extrusión26" cut sketch "Boceto33" against normal blind 32.3 contours A6 A0 | A0 A6 | A4 A0 | A0 A4 | A8 A0 | A0 A8 | A2 A0 | A0 A2 | A10 A0 | A0 A10 | A12 A0 | A0 A12
sketch "Boceto36" plane through (32.3, 0, 0) normal (1, 0, 0) x (0, 0, -1)
  circle A0 centre (0, 0) radius 3.5 projected
  circle A1 centre (0, 0) radius 28.5
  circle A2 centre (0, 0) radius 26
  circle A3 centre (0, 0) radius 26 projected
  circle A4 centre (0, 0) radius 28.5 projected
  constraints: 2 centre point, 2 coincident, 2 concentric
extrude "Extrusión27" cut sketch "Boceto36" against normal blind 2 contours A1
sketch "Boceto37" plane through (0, 0, 0) normal (-1, 0, 0) x (0, 0, 1)
  circle A0 centre (0, 0) radius 28.5
  circle A1 centre (0, 0) radius 26
  circle A2 centre (0, 0) radius 26 projected
  circle A3 centre (0, 0) radius 28.5 projected
  constraints: 2 centre point, 2 coincident, 2 concentric
extrude "Extrusión28" cut sketch "Boceto37" against normal blind 2
sketch "Boceto40" plane through (32.3, 0, 0) normal (1, 0, 0) x (0, 0, -1)
  circle A0 centre (0, 0) radius 19.25 construction
  arc A1 (17.3941, 12.637) -> (19.641, 8.7452) centre (18.6195, 10.75) ccw construction
  constraints: 1 centre point, 1 coincident, 1 tangent
